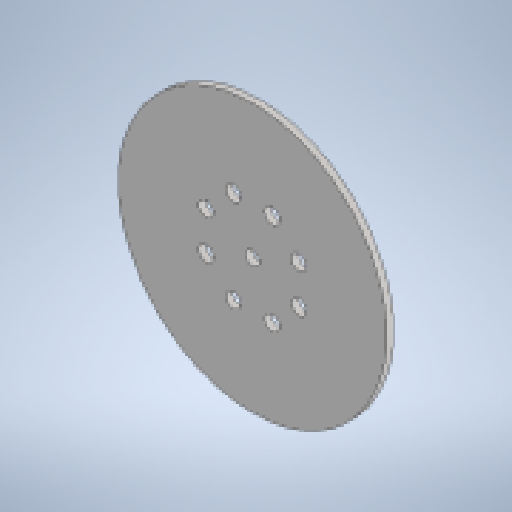
# Autodesk Inventor part: лицо
Saved by Autodesk Inventor 2023.1 (Build 271208000, 208)
## iProperties
Created: 2024-12-06
Part Number: лицо
Material: Типовые
Document SubType Name: Modeling
Designer: DELL
Density: 1 g/cm^3
Appearance: По умолчанию
Author: DELL
Autodesk Inventor part; units mm, degrees
ref_plane "YZ Plane" through (0, 0, 0) normal (1, 0, 0) x (0, 1, 0)
ref_plane "XZ Plane" through (0, 0, 0) normal (0, 1, 0) x (-1, 0, 0)
ref_plane "XY Plane" through (0, 0, 0) normal (0, 0, 1) x (1, 0, 0)
sketch "Эскиз1" plane through (0, 0, 0) normal (0, 0, 1) x (1, 0, 0)
  circle A0 centre (0, 0) radius 80 construction
  line L0 (76.2037, -11.1446) -> (61.4099, -21.4721) construction
  arc A1 (60.0176, -21.2246) -> (61.4099, -21.4721) centre (60.8375, -20.6521) ccw construction
  line L1 (60.0176, -21.2246) -> (37.9915, 10.3271) construction
  arc A2 (38.239, 11.7194) -> (37.9915, 10.3271) centre (38.8115, 10.8995) ccw construction
  line L2 (38.239, 11.7194) -> (53.0328, 22.0469) construction
  arc A3 (54.4252, 21.7994) -> (53.0328, 22.0469) centre (53.6052, 21.227) ccw construction
  line L3 (54.4252, 21.7994) -> (76.4513, -9.7522) construction
  arc A4 (76.2037, -11.1446) -> (76.4513, -9.7522) centre (75.6313, -10.3247) ccw construction
  circle A5 centre (0, 0) radius 80
  circle A6 centre (0, 0) radius 4 projected
  circle A7 centre (-27.7164, -11.4805) radius 4.5 projected
  circle A8 centre (27.7164, 11.4805) radius 4.5 projected
  circle A9 centre (-11.4805, 27.7164) radius 4.5 projected
  circle A10 centre (11.4805, -27.7164) radius 4.5 projected
  circle A11 centre (-11.4805, -27.7164) radius 4.5 projected
  circle A12 centre (-27.7164, 11.4805) radius 4.5 projected
  circle A13 centre (11.4805, 27.7164) radius 4.5 projected
  circle A14 centre (27.7164, -11.4805) radius 4.5 projected
  point P0 (0, 0)
  constraints: 1 centre point, 1 coincident, 1 concentric
extrude "Выдавливание1" add sketch "Эскиз1" along normal blind 4
